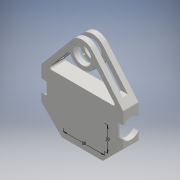
# Autodesk Inventor part: minibotv0.1
Saved by Autodesk Inventor 2016 (Build 200138000, 138)
## iProperties
Created: 2017-02-22
Part Number: minibotv0.1
Material: ABS Plastic
Document SubType Name: Modeling
Designer: Thomas
Mass: 51.8368 g
Surface Area: 283.459 cm^2
Volume: 48.9027 cm^3
Density: 1.06 g/cm^3
Appearance: Smooth - White
Author: Thomas
## iProperties of the stored document minibotv0.1_3DPrint.ipt
Created: 2017-02-23
Part Number: minibotv0.1_3DPrint
Material: Generic
Document SubType Name: Modeling
Designer: Thomas
Density: 1 g/cm^3
Appearance: Default
Author: Thomas
Autodesk Inventor part; units mm, degrees
ref_plane "YZ Plane" through (0, 0, 0) normal (1, 0, 0) x (0, 1, 0)
ref_plane "XZ Plane" through (0, 0, 0) normal (0, 1, 0) x (-1, 0, 0)
ref_plane "XY Plane" through (0, 0, 0) normal (0, 0, 1) x (1, 0, 0)
sketch "Sketch2" plane through (0, 0, 0) normal (0, 1, 0) x (-1, 0, 0)
  circle A0 centre (0, 0) radius 11
  line L0 (0, 0) -> (0, -148.579)
  line L1 (0, 0) -> (41.3171, -49.2398) construction
  line L2 (12.2567, 10.2846) -> (50, -34.6961)
  line L3 (50, -34.6961) -> (50, -74.6961)
  line L4 (41.8412, -34.6961) -> (0, -34.6961)
  line L5 (50, -74.6961) -> (25, -99.6961)
  line L6 (50, -74.6961) -> (85.3553, -74.6961) construction
  line L7 (25, -99.6961) -> (0, -99.6961)
  line L8 (-12.2567, 10.2846) -> (-50, -34.6961)
  line L9 (-50, -34.6961) -> (-50, -74.6961)
  line L10 (-41.8412, -34.6961) -> (0, -34.6961)
  line L11 (-50, -74.6961) -> (-25, -99.6961)
  line L12 (-25, -99.6961) -> (0, -99.6961)
  line L13 (-43.75, -40.9461) -> (-43.75, -72.1073)
  line L14 (-43.75, -72.1073) -> (-22.4112, -93.4461)
  line L15 (-22.4112, -93.4461) -> (0, -93.4461)
  line L16 (0, -93.4461) -> (22.4112, -93.4461)
  line L17 (22.4112, -93.4461) -> (43.75, -72.1073)
  line L18 (43.75, -72.1073) -> (43.75, -40.9461)
  line L19 (43.75, -40.9461) -> (0, -40.9461)
  line L20 (0, -40.9461) -> (-43.75, -40.9461)
  line L21 (15.6234, -3.4509) -> (41.8412, -34.6961)
  line L22 (-15.6234, -3.4509) -> (-41.8412, -34.6961)
  arc A1 (-15.6234, -3.4509) -> (15.6234, -3.4509) centre (0, 0) ccw
  arc A2 (12.2567, 10.2846) -> (-12.2567, 10.2846) centre (0, 0) ccw
  dimension "d4" = 22
  dimension "d6" = 40
  dimension "d7" = 100
  dimension "d8" = 40
  dimension "d9" = 135
  dimension "d10" = 50
  dimension "d11" = 6.25
  dimension "d12" = 6.25
  dimension "d15" = 6.25
  dimension "d16" = 6.25
  dimension "d17" = 6.25
  dimension "d18" = 6.25
  dimension "d19" = 16
  dimension "d20" = 90
  dimension "d21" = 40
  dimension "d22" = 25.4563
  dimension "d23" = 50
  dimension "d24" = 50
  dimension "d25" = 73.8829
  constraints: 46 end point, 4 parallel, 4 point on circle, 4 symmetric about line, 3 centre point, 3 horizontal, 2 coincident, 2 point on line, 2 tangent, 2 vertical, 1 equal length, 3 other
  measures "d4" diameter of A0
  measures "d6" angle of L0 L1
  measures "d7" diameter of L2.end L0
  measures "d8" distance of L2.end L3.end
  measures "d9" angle of L5 L6
  measures "d10" diameter of L5.end L0
  measures "d11" distance between parallel lines of L5 L17
  measures "d12" distance between parallel lines of L4 L19
  measures "d15" distance between parallel lines of L2 L21
  measures "d16" distance between parallel lines of L3 L18
  measures "d17" distance between parallel lines of L9 L13
  measures "d18" distance between parallel lines of L8 L22
  measures "d19" radius of A2
  measures "d20" angle of L10 L3
  measures "d21" distance between parallel lines of L4 L6
  measures "d22" distance from line of L1.end L6
  measures "d23" distance from line of L19.end L3
  measures "d24" distance from line of L15.end L3
  measures "d25" distance from line of L0.end L6
extrude "Extrusion2" add sketch "Sketch2" along normal blind 18.75
fillet "Fillet1" radius 2 10 edges at (15.6234, 9.375, -3.4509) (-15.6234, 9.375, -3.4509) (41.8412, 9.375, -34.6961) (-41.8412, 9.375, -34.6961) (50, 9.375, -34.6961) (-50, 9.375, -34.6961) (-50, 9.375, -74.6961) (-25, 9.375, -99.6961) (25, 9.375, -99.6961) (50, 9.375, -74.6961)
sketch "Sketch4" plane through (50, 0, -34.6961) normal (1, 0, 0) x (0, 0, -1)
  line L0 (-44.9807, 0) -> (-0.5576, 0) projected
  line L1 (-44.9807, 18.75) -> (-0.5576, 18.75) projected
  line L2 (-44.9807, 0) -> (-44.9807, 18.75) projected
  line L3 (-44.9807, 0) -> (-44.9807, 0) projected
  line L4 (-44.9807, 0) -> (-44.9807, 18.75) projected
  line L5 (-44.9807, 18.75) -> (-44.9807, 18.75) projected
  line L6 (-44.9807, 0) -> (-44.9807, 18.75) projected
  line L7 (-45.6961, 18.75) -> (-23.6961, 18.75) projected
  line L8 (-23.6961, 0) -> (-45.6961, 0) projected
  line L9 (0, 0) -> (0, 18.75) projected
  line L10 (0, 9.375) -> (-64.6192, 9.375) construction
  line L11 (-83.1961, 6.25) -> (-8.1961, 6.25)
  line L12 (-8.1961, 6.25) -> (-8.1961, 12.5)
  line L13 (-8.1961, 12.5) -> (-83.1961, 12.5)
  line L14 (-83.1961, 12.5) -> (-83.1961, 6.25)
  line L15 (-45.6961, 0) -> (-45.6961, 18.75) projected
  line L16 (-83.1961, 6.25) -> (-8.1961, 12.5) construction
  line L17 (-8.1961, 6.25) -> (-83.1961, 12.5) construction
  line L18 (-0.5576, 18.75) -> (-0.5576, 0) projected
  point P0 (-34.6961, 0)
  point P1 (-45.6961, 9.375)
  dimension "d30" = 75
  dimension "d31" = 6.25
  dimension "d34" = 6.25
  constraints: 14 end point, 4 midpoint, 2 parallel, 1 horizontal, 1 perpendicular
  measures "d30" distance of L11.start L11.end
  measures "d31" distance of L12.end L11.end
  measures "d34" distance from line of L1 L12.end
extrude "Extrusion3" cut sketch "Sketch4" against normal through all contours L11 L15 L13 L2 | L2 L13 L12 L11 | L11 L14 L13 L15
extrude "Extrusion4" add sketch "Sketch2" along normal blind 2 contours L19 L18 L17 L16 L0 | L0 L15 L14 L13 L20
sketch "Sketch5" plane through (50, 0, -35.424) normal (1, 0, 0) x (0, 0, -1)
  line L0 (5.5221, 2) -> (5.5221, 18.75) projected
  line L1 (5.5221, 2) -> (5.5221, 18.75) projected
  line L2 (38.4436, 18.75) -> (38.4436, 0) projected
  line L3 (0, 18.75) -> (38.4436, 18.75) projected
  line L4 (0, 0) -> (0, 18.75) projected
  line L5 (0, 0) -> (38.4436, 0) projected
  line L6 (36.6832, 2) -> (5.5221, 2) projected
  line L7 (58.0221, 2) -> (36.6832, 2) projected
  line L8 (5.5221, 2) -> (5.5221, 18.75) construction
  line L9 (5.5221, 18.75) -> (36.6832, 18.75) construction
  line L10 (5.5221, 2) -> (36.6832, 2) construction
  line L11 (5.5221, 9.375) -> (21.9828, 9.375) construction
  line L12 (21.9828, 9.375) -> (38.4436, 9.375) construction
  line L13 (38.4436, 18.75) -> (38.4436, 0) construction
  line L14 (21.9828, 9.375) -> (21.9828, 2)
  line L15 (21.9828, 9.375) -> (21.9828, 18.75) construction
  circle A0 centre (21.9828, 9.375) radius 10
  circle A1 centre (21.9828, 9.375) radius 12
  point P0 (-35.424, 0)
  dimension "d38" = 18.75
  dimension "d39" = 9.375
  dimension "d40" = 20
  dimension "d41" = 2
  constraints: 8 end point, 4 point on line, 2 centre point, 2 collinear, 2 perpendicular, 1 coincident, 1 midpoint, 1 vertical
  measures "d38" distance of L4.start L3.start
  measures "d39" distance from line of L3 point (21.983, 9.375)
  measures "d40" diameter of A0
  measures "d41" radial gap between concentric circles of A0 A1
extrude "Extrusion5" cut sketch "Sketch5" against normal up to surface (6.25 mm away) contours A1 L3 A0 L6 | L6 A0 L5 A1 | A1 L3 A0 | A0 L3 L6 | L6 A0 L5 | L5 A0 A1 | A0 L3 | A1 L6 A0 L3 | L5 A0 | L5 A0 L6 A1
mirror "Mirror1" about plane through (0, 0, 0) normal (1, 0, 0) of "Extrusion5"
sketch "Sketch6" plane through (43.75, 2, -47.9407) normal (1, 0, 0) x (0, 0, -1)
  line L0 (16.9568, -2) -> (1.9756, -2) projected
  arc A0 (16.9568, -2) -> (18.9324, 0) centre (9.4662, 7.375) ccw projected
  line L1 (18.9324, 0) -> (0, 0) projected
  arc A1 (0, 0) -> (1.9756, -2) centre (9.4662, 7.375) ccw projected
  line L2 (0.929, -0.125) -> (16.2419, -0.125) construction
  line L3 (-12.5166, -2) -> (1.9756, -2) projected
  line L4 (-12.5166, 16.75) -> (1.9756, 16.75) projected
  line L5 (1.9756, 7.375) -> (18.0034, 7.375) construction
  line L6 (9.4662, 7.375) -> (9.4662, -10.2466)
  line L7 (19.4662, 9.3155) -> (-0.5338, 9.3155)
  line L8 (-0.5338, 9.3155) -> (-0.5338, -0.125)
  line L9 (-0.5338, -0.125) -> (19.4662, -0.125)
  line L10 (19.4662, -0.125) -> (19.4662, 9.3155)
  line L11 (19.4662, 9.3155) -> (-0.5338, -0.125) construction
  line L12 (-0.5338, 9.3155) -> (19.4662, -0.125) construction
  point P0 (-47.9407, -2)
  point P1 (9.4662, 4.5953)
  dimension "d44" = 1.875
  dimension "d45" = 18.75
  dimension "d46" = 7.5
  dimension "d47" = 20
  constraints: 18 end point, 3 horizontal, 2 midpoint, 2 parallel, 2 point on line, 1 perpendicular, 1 vertical
  measures "d44" distance between parallel lines of L0 L2
  measures "d45" distance between parallel lines of L3 L4
  measures "d46" distance between parallel lines of L2 L5
  measures "d47" distance of L9.end L8.end
extrude "Extrusion6" cut sketch "Sketch6" against normal blind 36 contours L9 L6 L1 A0 | A0 L1 A1 L9 L8 L7 L10 | L9 A1 L1 L6
mirror "Mirror2" about plane through (0, 0, 0) normal (1, 0, 0) of "Extrusion6"
sketch "Sketch7" plane through (0, 2, 0) normal (0, 1, 0) x (1, 0, 0)
  line L0 (-25, 60.6941) -> (25, 60.6941)
  line L1 (25, 60.6941) -> (25, 90.6941)
  line L2 (25, 90.6941) -> (-25, 90.6941)
  line L3 (-25, 90.6941) -> (-25, 60.6941)
  line L4 (-25, 60.6941) -> (25, 90.6941) construction
  line L5 (25, 60.6941) -> (-25, 90.6941) construction
  point P0 (0, 0)
  point P1 (0, 75.6941)
  dimension "d50" = 50
  dimension "d51" = 30
  constraints: 12 end point, 2 midpoint, 2 parallel, 1 horizontal, 1 perpendicular
  measures "d50" distance of L2.end L1.end
  measures "d51" distance of L1.end L0.end
body "Solid2"
